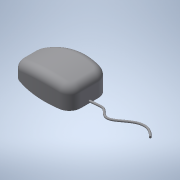
# Autodesk Inventor part: 06_03_Computer_Mouse
Saved by Autodesk Inventor 2020 (Build 240152000, 152)
## iProperties
Created: 2013-10-08
Part Number: 06_03_Computer_Mouse
Material: Generic
Document SubType Name: Modeling
Designer: John
Density: 1 g/cm^3
Appearance: Default
Author: John
Autodesk Inventor part; units mm, degrees
ref_plane "YZ Plane" through (0, 0, 0) normal (1, 0, 0) x (0, 1, 0)
sketch "Sketch1" plane through (0, 0, 0) normal (0, 0, 1) x (1, 0, 0)
  line L0 (0, 0) -> (101.6, 0)
  line L1 (101.6, 0) -> (101.6, 38.1)
  line L2 (101.6, 38.1) -> (0, 38.1)
  line L3 (0, 38.1) -> (0, 0)
  arc A0 (101.6, 31.9501) -> (0, 19.05) centre (64.1041, -79.2816) ccw
  dimension "d0" = 101.6
  dimension "d1" = 38.1
  constraints: 8 end point, 2 parallel, 2 point on circle, 1 centre point, 1 horizontal, 1 midpoint, 1 perpendicular, 1 point on line, 1 tangent
  measures "d0" distance of L2.end L1.end
  measures "d1" distance of L1.end L0.end
extrude "Extrusion1" add sketch "Sketch1" along normal mid plane 69.85 contours L3 A0 L1 L0
sketch "Sketch2" plane through (0, 0, 34.925) normal (0, -1, 0) x (1, 0, 0)
  line L0 (101.6, -69.85) -> (101.6, 0) projected
  line L1 (0, 0) -> (101.6, 0) projected
  line L2 (0, 0) -> (0, -69.85) projected
  line L3 (101.6, -69.85) -> (0, -69.85) projected
  arc A0 (101.6, -5.0773) -> (0, -13.4171) centre (62.5658, -152.5848) ccw
  point P0 (0, -34.925)
  constraints: 2 point on circle, 2 point on line, 1 centre point, 1 tangent
extrude "Extrusion2" cut sketch "Sketch2" against normal through all contours A0 L1 L0 | A0 L2 L1
mirror "Mirror1" about plane through (0, 0, 0) normal (0, 0, 1) of "Extrusion2"
fillet "Fillet1" radius 19.05 4 edges at (101.6, 15.9751, 29.8477) (101.6, 15.9751, -29.8477) (0, 9.525, -21.5079) (0, 9.525, 21.5079)
fillet "Fillet2" radius 12.7 10 edges at (35.9307, 34.6688, 32.5823) (74.1438, 37.6699, 34.4851) (97.6991, 33.1898, 25.9214) (101.6, 31.9501, 0) (97.6991, 33.1898, -25.9214) (74.1438, 37.6699, -34.4851) (35.9307, 34.6688, -32.5823) (3.3248, 21.1391, -19.3384) (0, 19.05, 0) (3.3248, 21.1391, 19.3384)
ref_plane "Work Plane1" through (101.6, 3.175, -14.3712) normal (0, -1, 0) x (1, 0, 0)
sketch "Sketch3" plane through (101.6, 3.175, -14.3712) normal (0, -1, 0) x (1, 0, 0)
  line L0 (-5.1165, 14.3712) -> (20.8176, 14.3712) construction
  line L1 (20.8176, 14.3712) -> (23.4549, 0.525) construction
  line L2 (23.4549, 0.525) -> (37.5209, 62.0635) construction
  line L3 (37.5209, 62.0635) -> (72.9055, -15.5189) construction
  line L4 (72.9055, -15.5189) -> (101.9165, 16.1294) construction
  spline S0 degree 4 poles (-5.1165, 14.3712) (20.8176, 14.3712) (23.4549, 0.525) (37.5209, 62.0635) (72.9055, -15.5189) (101.9165, 16.1294) knots 1 1 1 1 1 2 3 3 3 3 3
  point P0 (-101.6, 14.3712)
  constraints: 1 horizontal, 3 other
ref_plane "Work Plane2" through (96.4835, 3.175, 0) normal (1, 0, 0) x (0, 1, 0)
sketch "Sketch4" plane through (96.4835, 3.175, 0) normal (1, 0, 0) x (0, 1, 0)
  circle A0 centre (0, 0) radius 1.5875
  point P0 (-3.175, 0)
  dimension "d9" = 3.175
  constraints: 1 centre point
  measures "d9" diameter of A0
sweep "Sweep1" add profiles "Sketch4" path "Sketch3"
body "Solid1"
